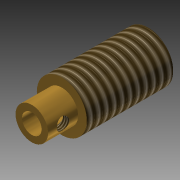
# Autodesk Inventor part: Worm Gear
Saved by Autodesk Inventor 2015 SP1 (Build 190203100, 203)
## iProperties
Created: 2015-02-24
Part Number: Worm Gear
Material: Brass, Soft Yellow
Document SubType Name: Modeling
Designer: Andrew
Density: 8.47 g/cm^3
Appearance: Brass - Satin
Author: Andrew
Autodesk Inventor part; units mm, degrees
ref_plane "YZ Plane" through (0, 0, 0) normal (1, 0, 0) x (0, 1, 0)
ref_plane "XZ Plane" through (0, 0, 0) normal (0, 1, 0) x (-1, 0, 0)
ref_plane "XY Plane" through (0, 0, 0) normal (0, 0, 1) x (1, 0, 0)
sketch "Sketch1" plane through (0, 0, 0) normal (0, 1, 0) x (-1, 0, 0)
  circle A0 centre (0, 0) radius 4.1275
  circle A1 centre (0, 0) radius 6.35
  dimension "d0" = 12.7
  dimension "d1" = 8.255
  constraints: 2 centre point, 2 coincident
  measures "d0" diameter of A1
  measures "d1" diameter of A0
extrude "Extrusion1" add sketch "Sketch1" along normal blind 21.925 contours A0 | A1
extrude "Extrusion2" add sketch "Sketch1" against normal blind 7.62 contours A0
sketch "Sketch2" plane through (0, -7.62, 0) normal (0, -1, 0) x (1, 0, 0)
  circle A0 centre (0, 0) radius 2.5
  dimension "d6" = 5
  constraints: 1 centre point, 1 coincident
  measures "d6" diameter of A0
extrude "Extrusion3" cut sketch "Sketch2" against normal up to next
thread "Thread1" size "M14x2" class "6g" standard "ANSI Metric M Profile" full length
sketch "Sketch3" plane through (0, 0, 0) normal (1, 0, 0) x (0, 1, 0)
  line L0 (-13.529, 0) -> (27.834, 0) projected
  line L1 (0, 8.89) -> (0, -8.89) projected
  circle A0 centre (-3.81, 0) radius 1.5875
  line L2 (-7.62, -2.5) -> (-7.62, 2.5) projected
  line L3 (0, 4.1275) -> (-7.62, 4.1275) construction
  line L4 (-3.81, 4.1275) -> (-3.81, -2.5) construction
  point P0 (0, 0)
  dimension "d11" = 3.175
  constraints: 2 end point, 2 point on line, 1 centre point, 1 midpoint, 1 vertical
  measures "d11" diameter of A0
extrude "Extrusion4" cut sketch "Sketch3" along normal up to surface round surface about axis through (0, 0, 0) along (0, -1, 0) radius 4.1275 far side no
thread "Thread2" size "M3.5x0.6" class "6H" standard "ANSI Metric M Profile" full length
body "Solid1"
